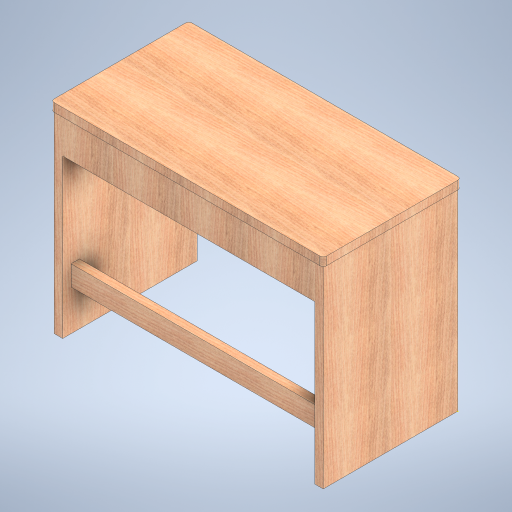
# Autodesk Inventor part: Desk
Saved by Autodesk Inventor 2023 (Build 270158000, 158)
## iProperties
Created: 2022-09-17
Part Number: Desk
Material: Wood (Birch)
Document SubType Name: Modeling
Designer: mliu-23
Density: 0.55 g/cm^3
Appearance: Birch - Natural Polished
Author: mliu-23
Autodesk Inventor part; units mm, degrees
ref_plane "YZ Plane" through (0, 0, 0) normal (1, 0, 0) x (0, 1, 0)
ref_plane "XZ Plane" through (0, 0, 0) normal (0, 1, 0) x (-1, 0, 0)
sketch "Sketch1" plane through (0, 0, 0) normal (0, 1, 0) x (-1, 0, 0)
  point P0 (0, 0)
sketch "Sketch2" plane through (0, 0, 0) normal (0, 1, 0) x (-1, 0, 0)
  line L0 (0, 0) -> (1016, 0)
  line L1 (1016, 0) -> (1016, 508)
  line L2 (1016, 508) -> (0, 508)
  line L3 (0, 508) -> (0, 0)
  line L4 (0, 508) -> (31.75, 508)
  line L5 (31.75, 508) -> (31.75, 0)
  line L6 (31.75, 0) -> (0, 0)
  line L7 (0, 0) -> (0, 508)
  line L8 (1016, 508) -> (984.25, 508)
  line L9 (984.25, 508) -> (984.25, 0)
  line L10 (984.25, 0) -> (1016, 0)
  line L11 (1016, 0) -> (1016, 508)
  dimension "d0" = 1016
  dimension "d1" = 508
  dimension "d2" = 31.75
  dimension "d3" = 31.75
  constraints: 24 end point, 6 parallel, 3 horizontal, 3 perpendicular, 2 point on line
  measures "d0" distance of L2.end L1.end
  measures "d1" distance of L1.end L0.end
  measures "d2" distance of L5.end L6.end
  measures "d3" distance of L10.end L9.end
extrude "Extrusion1" add sketch "Sketch2" along normal blind 730.25 contours L3 L2 L5 L0 | L9 L2 L1 L0
sketch "Sketch3" plane through (0, 730.25, 0) normal (0, 1, 0) x (1, 0, 0)
  line L0 (0, -508) -> (0, 0) projected
  line L1 (-1016, 0) -> (-1016, -508) projected
  line L2 (0, 0) -> (-1016, 0)
  line L3 (-1016, 0) -> (-1016, -508)
  line L4 (-1016, -508) -> (0, -508)
  line L5 (0, -508) -> (0, 0)
  line L6 (-1022.35, 6.35) -> (6.35, 6.35)
  line L7 (6.35, 6.35) -> (6.35, -514.35)
  line L8 (6.35, -514.35) -> (-1022.35, -514.35)
  line L9 (-1022.35, -514.35) -> (-1022.35, 6.35)
  dimension "d6" = 6.35
  constraints: 16 end point, 4 parallel, 2 perpendicular, 1 horizontal, 3 other
  measures "d6" distance between parallel lines of L2 L6
extrude "Extrusion2" add sketch "Sketch3" along normal blind 31.75 contours L4 L1 L2 L0 | L6 L7 L8 L9
sketch "Sketch4" plane through (0, 730.25, 0) normal (0, -1, 0) x (1, 0, 0)
  line L0 (-984.25, 508) -> (-984.25, 0) projected
  line L1 (-31.75, 508) -> (-984.25, 508)
  line L2 (-984.25, 508) -> (-984.25, 38.1)
  line L3 (-984.25, 38.1) -> (-31.75, 38.1)
  line L4 (-31.75, 38.1) -> (-31.75, 508)
  point P0 (0, 0)
  dimension "d9" = 469.9
  constraints: 8 end point, 2 parallel, 1 horizontal, 1 perpendicular, 1 point on line
  measures "d9" distance from line of L3 L1.end
extrude "Extrusion3" add sketch "Sketch4" along normal blind 31.75
fillet "Fillet1" radius 12.7 4 edges at (6.35, 746.125, -6.35) (-1022.35, 746.125, -6.35) (-1022.35, 746.125, 514.35) (6.35, 746.125, 514.35)
sketch "Sketch5" plane through (-31.75, 0, 0) normal (-1, 0, 0) x (0, 0, 1)
  line L0 (0, 0) -> (0, 730.25) projected
  line L1 (508, 0) -> (508, 730.25) projected
  line L2 (0, 577.85) -> (508, 577.85)
  line L3 (508, 577.85) -> (508, 546.1)
  line L4 (508, 546.1) -> (0, 546.1)
  line L5 (0, 546.1) -> (0, 577.85)
  line L6 (0, 730.25) -> (38.1, 730.25) projected
  line L7 (152.4, 577.85) -> (152.4, 546.1)
  line L8 (254, 577.85) -> (254, 546.1)
  point P0 (0, 546.1)
  dimension "d13" = 152.4
  dimension "d14" = 31.75
  dimension "d17" = 152.4
  constraints: 12 end point, 4 point on line, 2 midpoint, 2 parallel, 2 perpendicular, 1 horizontal
  measures "d13" distance between parallel lines of L6 L2
  measures "d14" distance between parallel lines of L4 L2
  measures "d17" distance between parallel lines of L0 L7
extrude "Extrusion4" add sketch "Sketch5" along normal up to surface (952.5 mm away) contours L7 L2 L8 L4
sketch "Sketch6" plane through (-31.75, 0, 0) normal (-1, 0, 0) x (0, 0, 1)
  line L0 (0, 0) -> (508, 0) projected
  line L1 (508, 0) -> (508, 730.25) projected
  line L2 (0, 730.25) -> (508, 730.25) projected
  line L3 (0, 0) -> (0, 730.25) projected
  line L4 (6.35, 730.25) -> (501.65, 730.25) projected
  line L5 (444.5, 228.6) -> (476.25, 228.6)
  line L6 (476.25, 228.6) -> (476.25, 152.4)
  line L7 (476.25, 152.4) -> (444.5, 152.4)
  line L8 (444.5, 152.4) -> (444.5, 228.6)
  point P0 (476.25, 190.5)
  dimension "d18" = 31.75
  dimension "d19" = 76.2
  dimension "d20" = 31.75
  dimension "d21" = 152.4
  constraints: 8 end point, 2 parallel, 1 horizontal, 1 midpoint, 1 perpendicular
  measures "d18" distance of L6.end L7.end
  measures "d19" distance of L5.end L6.end
  measures "d20" distance from line of L1 point (476.25, 190.5)
  measures "d21" distance between parallel lines of L0 L7
extrude "Extrusion5" add sketch "Sketch6" along normal up to surface (952.5 mm away) contours L5 L6 L7 L8
sketch "Sketch7" plane through (-31.75, 0, 0) normal (-1, 0, 0) x (0, 0, 1)
  line L0 (508, 698.5) -> (38.1, 698.5) projected
  line L1 (508, 698.5) -> (476.25, 698.5)
  line L2 (476.25, 698.5) -> (476.25, 596.9)
  line L3 (476.25, 596.9) -> (508, 596.9)
  line L4 (508, 596.9) -> (508, 698.5)
  point P0 (0, 0)
  dimension "d24" = 31.75
  dimension "d25" = 101.6
  constraints: 8 end point, 2 parallel, 1 horizontal, 1 perpendicular
  measures "d24" distance of L3.end L2.end
  measures "d25" distance of L2.end L1.end
extrude "Extrusion6" add sketch "Sketch7" along normal up to surface (952.5 mm away)
sketch "Sketch8" plane through (-31.75, 0, 0) normal (-1, 0, 0) x (0, 0, 1)
  line L0 (476.25, 596.9) -> (476.25, 698.5) projected
  line L1 (0, 635) -> (476.25, 635)
  line L2 (476.25, 635) -> (476.25, 596.9)
  line L3 (476.25, 596.9) -> (0, 596.9)
  line L4 (0, 596.9) -> (0, 635)
  line L5 (0, 0) -> (0, 730.25) projected
  dimension "d28" = 38.1
  constraints: 8 end point, 2 parallel, 1 collinear, 1 horizontal, 1 perpendicular
  measures "d28" distance between parallel lines of L3 L1
extrude "Extrusion7" add sketch "Sketch8" along normal blind 19.05 separate body
ref_plane "Work Plane1" through (-508, 0, 0) normal (-1, 0, 0) x (0, 0, 1)
mirror "Mirror1" about plane through (-508, 0, 0) normal (-1, 0, 0) of "Extrusion7" bodies 2
body "Solid1"
body "Solid2"
